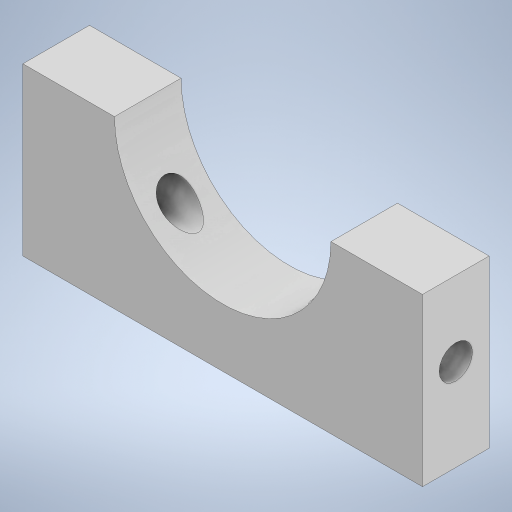
# Autodesk Inventor part: Frame Bottom
Saved by Autodesk Inventor 2023 (Build 270158000, 158)
## iProperties
Created: 2022-10-29
Part Number: Frame Bottom
Material: Generic
Document SubType Name: Modeling
Designer: tommy
Density: 1 g/cm^3
Appearance: Default
Author: tommy
Autodesk Inventor part; units mm, degrees
ref_plane "YZ Plane" through (0, 0, 0) normal (1, 0, 0) x (0, 1, 0)
ref_plane "XZ Plane" through (0, 0, 0) normal (0, 1, 0) x (-1, 0, 0)
ref_plane "XY Plane" through (0, 0, 0) normal (0, 0, 1) x (1, 0, 0)
sketch "Sketch1" plane through (0, 0, 0) normal (0, 0, 1) x (1, 0, 0)
  arc A0 (20.6801, 49.5146) -> (61.9551, 49.5146) centre (41.3176, 49.5146) ccw
  line L0 (3.2176, 49.5146) -> (79.4176, 49.5146)
  line L1 (3.2176, 49.5146) -> (3.2176, 17.7646)
  line L2 (79.4176, 49.5146) -> (79.4176, 17.7646)
  line L3 (79.4176, 17.7646) -> (3.2176, 17.7646)
  dimension "d21" = 31.75
  dimension "d22" = 31.75
  constraints: 8 end point, 2 point on circle, 2 point on line, 2 vertical, 1 centre point, 1 horizontal, 1 midpoint
  measures "d21" distance of L0.start L1.end
  measures "d22" distance of L0.end L2.end
extrude "Extrusion4" add sketch "Sketch1" along normal blind 12.7 contours A0 L0 L2 L3 L1
sketch "Sketch2" plane through (79.4176, 17.7646, 0) normal (1, 0, 0) x (0, 0, -1)
  line L0 (0, 31.75) -> (-12.7, 31.75) projected
  circle A0 centre (-6.35, 17.4498) radius 3.175
  point P0 (0, -17.7646)
  dimension "d26" = 6.35
  constraints: 1 centre point
  measures "d26" diameter of A0
extrude "Extrusion5" cut sketch "Sketch2" against normal blind 96.8375
body "Solid4"
